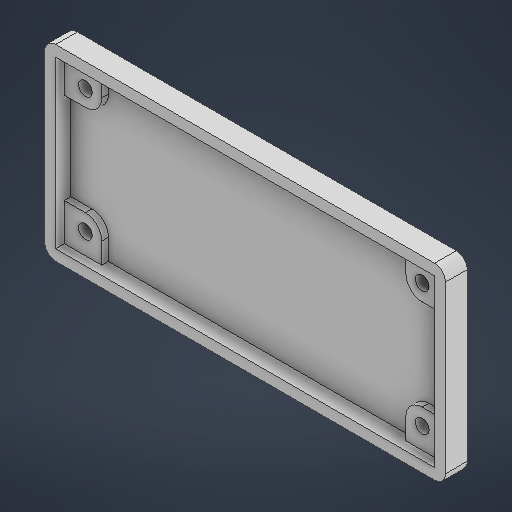
# Autodesk Inventor part: power_sync_module_case
Saved by Autodesk Inventor 2026 (Build 300175000, 175)
## iProperties
Created: 2026-03-10
Part Number: power_sync_module_case
Material: Generic
Document SubType Name: Modeling
Designer: numai
Density: 1 g/cm^3
Appearance: Default
Author: numai
Autodesk Inventor part; units mm, degrees
ref_plane "YZ Plane" through (0, 0, 0) normal (1, 0, 0) x (0, 1, 0)
ref_plane "XZ Plane" through (0, 0, 0) normal (0, 1, 0) x (-1, 0, 0)
ref_plane "XY Plane" through (0, 0, 0) normal (0, 0, 1) x (1, 0, 0)
sketch "スケッチ1" plane through (0, 0, 0) normal (0, 0, 1) x (1, 0, 0)
  line L0 (-34.7, 15.2) -> (34.7, 15.2)
  line L1 (34.7, 15.2) -> (34.7, -15.2)
  line L2 (34.7, -15.2) -> (-34.7, -15.2)
  line L3 (-34.7, -15.2) -> (-34.7, 15.2)
  line L4 (-30.85, 11.35) -> (30.85, 11.35) construction
  line L5 (30.85, 11.35) -> (30.85, -11.35) construction
  line L6 (30.85, -11.35) -> (-30.85, -11.35) construction
  line L7 (-30.85, -11.35) -> (-30.85, 11.35) construction
  circle A0 centre (-30.85, 11.35) radius 1.25
  circle A1 centre (-30.85, -11.35) radius 1.25
  circle A2 centre (30.85, -11.35) radius 1.25
  circle A3 centre (30.85, 11.35) radius 1.25
  line L8 (36.7, 17.2) -> (-36.7, 17.2)
  line L9 (-36.7, 17.2) -> (-36.7, -17.2)
  line L10 (-36.7, -17.2) -> (36.7, -17.2)
  line L11 (36.7, -17.2) -> (36.7, 17.2)
  point P0 (0, 0)
  point P1 (0, 15.2)
  point P2 (-34.7, 0)
  point P3 (0, 11.35)
  point P4 (-30.85, 0)
  dimension "d0" = 30.4
  dimension "d1" = 69.4
  dimension "d2" = 61.7
  dimension "d3" = 22.7
  dimension "d4" = 2.5
  dimension "d5" = 2
  constraints: 24 end point, 6 parallel, 4 centre point, 4 coincident, 4 midpoint, 3 equal radius, 3 perpendicular, 2 horizontal, 2 horizontal alignment, 2 vertical alignment, 3 other
  measures "d0" distance of L2.end L0.start
  measures "d1" distance of L0.start L0.end
  measures "d2" distance of L4.start L4.end
  measures "d3" distance of L6.end L4.start
  measures "d4" diameter of A0
  measures "d5" distance between parallel lines of L0 L8
extrude "押し出し1" add sketch "スケッチ1" along normal blind 1.6 contours L11 L10 L9 L8
extrude "押し出し2" add sketch "スケッチ1" against normal blind 2.4 contours L0 L1 L2 L3 | L11 L10 L9 L8
sketch "スケッチ2" plane through (0, 0, 0) normal (0, 0, 1) x (1, 0, 0)
  circle A0 centre (-30.85, -11.35) radius 1.25 construction
  circle A1 centre (-30.85, 11.35) radius 1.25 construction
  circle A2 centre (30.85, -11.35) radius 1.25 construction
  circle A3 centre (30.85, 11.35) radius 1.25 construction
  line L0 (-34.7, -15.2) -> (-34.7, 15.2) projected
  line L1 (34.7, -15.2) -> (-34.7, -15.2) projected
  line L2 (-34.7, 15.2) -> (34.7, 15.2) projected
  line L3 (34.7, 15.2) -> (34.7, -15.2) projected
  line L4 (-27.85, -15.2) -> (-27.85, -11.35)
  arc A4 (-27.85, -11.35) -> (-30.85, -8.35) centre (-30.85, -11.35) ccw
  line L5 (-30.85, -8.35) -> (-34.7, -8.35)
  line L6 (-34.7, 8.35) -> (-30.85, 8.35)
  arc A5 (-30.85, 8.35) -> (-27.85, 11.35) centre (-30.85, 11.35) ccw
  line L7 (-27.85, 11.35) -> (-27.85, 15.2)
  line L8 (27.85, -15.2) -> (27.85, -11.35)
  arc A6 (30.85, -8.35) -> (27.85, -11.35) centre (30.85, -11.35) ccw
  line L9 (30.85, -8.35) -> (34.7, -8.35)
  line L10 (34.7, 8.35) -> (30.85, 8.35)
  arc A7 (27.85, 11.35) -> (30.85, 8.35) centre (30.85, 11.35) ccw
  line L11 (27.85, 11.35) -> (27.85, 15.2)
  point P0 (0, 0)
  dimension "d10" = 3
  constraints: 16 end point, 8 point on circle, 8 point on line, 8 tangent, 4 centre point, 4 concentric, 4 perpendicular, 3 equal radius, 2 horizontal, 2 vertical
  measures "d10" radius of A4
extrude "押し出し3" cut sketch "スケッチ2" against normal blind 1.2 contours L0 L6 A5 L7 L2 L11 A7 L10 L3 L9 A6 L8 L1 L4 A4 L5
fillet "フィレット1" radius 2 4 edges at (-36.7, 17.2, -0.4) (-36.7, -17.2, -0.4) (36.7, -17.2, -0.4) (36.7, 17.2, -0.4)
